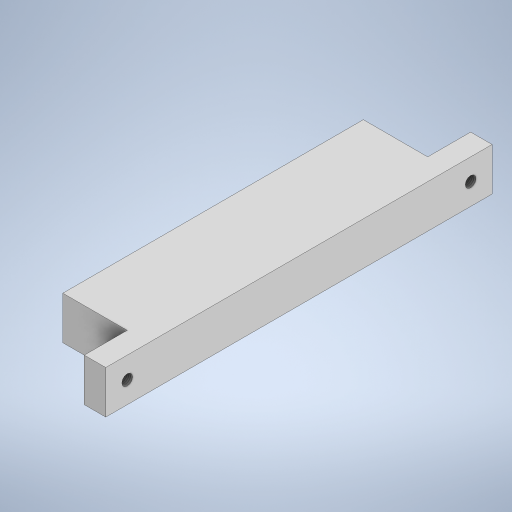
# Autodesk Inventor part: Подставка подшипника
Saved by Autodesk Inventor 2023 (Build 270158000, 158)
## iProperties
Created: 2022-05-17
Part Number: Подставка подшипника
Material: Типовые
Document SubType Name: Modeling
Designer: avkap
Density: 1 g/cm^3
Appearance: По умолчанию
Author: avkap
Autodesk Inventor part; units mm, degrees
ref_plane "YZ Plane" through (0, 0, 0) normal (1, 0, 0) x (0, 1, 0)
ref_plane "XZ Plane" through (0, 0, 0) normal (0, 1, 0) x (-1, 0, 0)
ref_plane "XY Plane" through (0, 0, 0) normal (0, 0, 1) x (1, 0, 0)
sketch "Эскиз1" plane through (0, 0, 0) normal (0, 1, 0) x (-1, 0, 0)
  line L0 (0, 0) -> (10, 0)
  line L1 (10, 0) -> (10, -20)
  line L2 (10, -20) -> (40, -20)
  line L3 (40, -20) -> (40, -160)
  line L4 (40, -160) -> (10, -160)
  line L5 (10, -160) -> (10, -180)
  line L6 (10, -180) -> (0, -180)
  line L7 (0, -180) -> (0, 0)
  line L8 (40, -160) -> (35, -160)
  line L9 (40, -150) -> (40, -130)
  line L10 (40, -20) -> (35, -20)
  line L11 (40, -30) -> (40, -50)
  line L12 (40, -90) -> (35, -90)
  line L13 (35, -90) -> (35, -123)
  line L14 (35, -123) -> (40, -123)
  line L15 (35, -90) -> (35, -57)
  line L16 (35, -57) -> (40, -57)
  line L17 (40, -123) -> (40, -133)
  line L18 (40, -133) -> (35, -133)
  line L19 (35, -133) -> (35, -160)
  line L20 (40, -57) -> (40, -47)
  line L21 (40, -47) -> (35, -47)
  line L22 (35, -47) -> (35, -20)
  point P0 (40, -47)
  dimension "d0" = 10
  dimension "d1" = 20
  dimension "d2" = 30
  dimension "d3" = 140
  dimension "d4" = 20
  dimension "d54" = 33
  dimension "d55" = 33
  dimension "d56" = 10
  dimension "d57" = 10
  constraints: 44 end point, 8 perpendicular, 8 point on line, 5 horizontal, 1 vertical, 10 other
  measures "d0" distance of L0.start L0.end
  measures "d1" distance of L0.end L1.end
  measures "d2" distance of L1.end L2.end
  measures "d3" distance of L2.end L4.start
  measures "d4" distance of L4.end L5.end
  measures "d54" distance of L12.end L13.end
  measures "d55" distance of L12.end L15.end
  measures "d56" distance of L14.end L17.end
  measures "d57" distance of L16.end L20.end
extrude "Выдавливание1" add sketch "Эскиз1" along normal blind 20
sketch "Эскиз2" plane through (-10, 0, -20) normal (-1, 0, 0) x (0, 0, 1)
  line L0 (0, 0) -> (20, 0) projected
  line L1 (20, 0) -> (0, 0)
  line L2 (0, 0) -> (10, 0)
  line L3 (10, 0) -> (10, 10)
  line L4 (20, 20) -> (-160, 20) projected
  line L5 (10, 20) -> (10, 10)
  line L6 (-140, 0) -> (-140, 20) projected
  line L7 (-160, 20) -> (-140, 20)
  line L8 (-140, 20) -> (-150, 20)
  line L9 (-150, 20) -> (-150, 10)
  line L10 (-150, 0) -> (-150, 10)
  circle A0 centre (10, 10) radius 2.5
  circle A1 centre (-150, 10) radius 2.5
  dimension "d7" = 10
  dimension "d10" = 10
  dimension "d12" = 5
  dimension "d14" = 5
  constraints: 16 end point, 6 point on line, 3 perpendicular, 2 centre point, 2 coincident, 2 midpoint, 1 horizontal
  measures "d7" distance of L2.end L3.end
  measures "d10" distance of L10.start L10.end
  measures "d12" diameter of A0
  measures "d14" diameter of A1
extrude "Выдавливание2" cut sketch "Эскиз2" against normal blind 44.25
thread "Резьба4" size "M5x0.8" class "6H" standard "ANSI Metric M Profile" full length
sketch "Эскиз3" plane through (-40, 0, -160) normal (-1, 0, 0) x (0, 0, 1)
  line L0 (140, 0) -> (140, 20) projected
  line L1 (140, 0) -> (140, 10)
  line L2 (140, 0) -> (70, 0)
  line L3 (160, 0) -> (-20, 0) projected
  line L4 (70, 10) -> (120, 10)
  line L5 (120, 10) -> (20, 10)
  line L6 (70, 10) -> (70, 0)
  circle A0 centre (120, 10) radius 5
  circle A1 centre (20, 10) radius 5
  line L7 (120, 10) -> (140, 10)
  dimension "d28" = 50
  dimension "d29" = 100
  dimension "d30" = 10
  dimension "d31" = 10
  dimension "d41" = 10
  dimension "d48" = 20
  constraints: 12 end point, 2 centre point, 2 coincident, 2 horizontal, 2 midpoint, 1 perpendicular
  measures "d28" distance of L4.start L4.end
  measures "d29" distance of L4.end L5.end
  measures "d30" diameter of A0
  measures "d31" diameter of A1
  measures "d41" distance of L4.start L2.end
  measures "d48" distance of L7.start L1.end
extrude "Выдавливание3" cut sketch "Эскиз3" against normal blind 20 contours L7 L4 A0 | A0 L4 L7 | A1
thread "Резьба7" size "M5x0.8" class "6H" standard "ANSI Metric M Profile" full length
thread "Резьба8" size "M10x1.5" class "6H" standard "ANSI Metric M Profile" full length
thread "Резьба9" size "M10x1.5" class "6H" standard "ANSI Metric M Profile" full length
